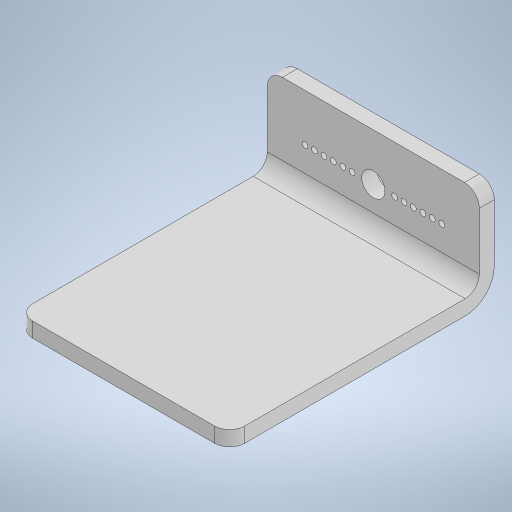
# Autodesk Inventor part: Platform
Saved by Autodesk Inventor 2023.4 (Build 274418000, 418)
## iProperties
Created: 2024-05-24
Part Number: Platform
Material: Generic
Document SubType Name: Modeling
Designer: Nathan Cai
Mass: 10.221 g
Surface Area: 73.6667 cm^2
Volume: 10.221 cm^3
Density: 1 g/cm^3
Appearance: Default
Author: Nathan Cai
Autodesk Inventor part; units mm, degrees
note: some values were not read from the file. Chosen so that the rebuilt part matches the saved one: bend side of "Bend Part1".
ref_plane "YZ Plane" through (0, 0, 0) normal (1, 0, 0) x (0, 1, 0)
ref_plane "XZ Plane" through (0, 0, 0) normal (0, 1, 0) x (-1, 0, 0)
ref_plane "XY Plane" through (0, 0, 0) normal (0, 0, 1) x (1, 0, 0)
sketch "Sketch1" plane through (0, 0, 0) normal (0, 1, 0) x (-1, 0, 0)
  line L0 (22.5, 35) -> (-22.5, 35)
  line L1 (-22.5, 35) -> (-22.5, -35)
  line L2 (-22.5, -35) -> (22.5, -35)
  line L3 (22.5, -35) -> (22.5, 35)
  line L4 (22.5, 35) -> (-22.5, -35) construction
  line L5 (-22.5, 35) -> (22.5, -35) construction
  line L6 (0, 0) -> (0, -35) construction
  circle A0 centre (0, -25) radius 2.5
  circle A1 centre (0, -25) radius 4.5 construction
  line L7 (0, -25) -> (-4.5, -25) construction
  circle A2 centre (-4.5, -25) radius 0.625
  circle A3 centre (-6.5, -25) radius 0.625
  circle A4 centre (-8.5, -25) radius 0.625
  circle A5 centre (-10.5, -25) radius 0.625
  circle A6 centre (-12.5, -25) radius 0.625
  circle A7 centre (-14.5, -25) radius 0.625
  circle A8 centre (4.5, -25) radius 0.625
  circle A9 centre (6.5, -25) radius 0.625
  circle A10 centre (8.5, -25) radius 0.625
  circle A11 centre (10.5, -25) radius 0.625
  circle A12 centre (12.5, -25) radius 0.625
  circle A13 centre (14.5, -25) radius 0.625
  dimension "d3" = 9
  dimension "d0" = 45
  dimension "d1" = 70
  dimension "d2" = 5
  dimension "d4" = 1.25
  dimension "d7" = 2
  dimension "d14" = 360
  dimension "d16" = 10
  constraints: 16 end point, 13 centre point, 3 coincident, 3 horizontal, 3 midpoint, 2 parallel, 1 horizontal alignment, 1 perpendicular, 1 point on line, 39 other
  measures "d0" distance of L2.end L1.end
  measures "d1" distance of L1.end L0.end
  measures "d2" diameter of A0
  measures "d4" diameter of A2
  measures "d7" distance of A2.centre A3.centre
  measures "d16" distance from line of L2 A0.centre
extrude "Extrusion1" add sketch "Sketch1" along normal blind 3.175
fillet "Fillet1" radius 3.175 4 edges at (22.5, 1.5875, -35) (-22.5, 1.5875, -35) (-22.5, 1.5875, 35) (22.5, 1.5875, 35)
sketch "Sketch2" plane through (0, 3.175, 0) normal (0, 1, 0) x (1, 0, 0)
  line L0 (-22.5, 31.825) -> (-22.5, -31.825) projected
  line L1 (-22.5, 15) -> (22.5, 15)
  line L2 (22.5, -31.825) -> (22.5, 31.825) projected
  line L3 (19.325, 35) -> (-19.325, 35) projected
  point P0 (0, 0)
  dimension "d20" = 20
  constraints: 2 end point, 2 point on line, 1 horizontal
  measures "d20" distance between parallel lines of L3 L1
bend part "Bend Part1" radius 3 angle 90 line through (-22.5, 3.175, -15) along (1, 0, 0) centre toward (0, 1, 0) moving side (0, 0, -1) both sides no
body "Solid1"
